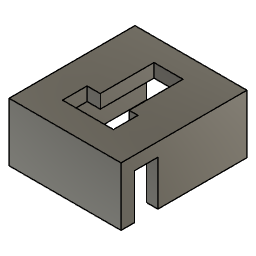
SNES - Back Cutting Tool v11 (Autodesk Fusion 360 design; units mm, degrees)
Autodesk Fusion 360 part; units mm, degrees
note: some values were not read from the file. Set by a fixed rule: which sketch regions a step uses.
sketch "Boceto1" plane through (0, 0, 0) normal (0, 0, 1) x (1, 0, 0)
  line L0 (4.725, 2.765) -> (4.725, -5.635)
  line L1 (4.725, -8.235) -> (-4.725, -8.235)
  line L2 (-4.725, -8.235) -> (-4.725, 2.765)
  line L3 (-6.225, 4.265) -> (6.225, 4.265)
  line L4 (6.225, 4.265) -> (6.225, -9.735)
  line L5 (6.225, -9.735) -> (-6.225, -9.735)
  line L6 (-6.225, -9.735) -> (-6.225, 4.265)
  line L7 (2.585, -4.215) -> (2.585, -6.945)
  line L8 (2.585, -6.945) -> (-3.075, -6.945)
  line L9 (-3.075, -6.945) -> (-3.075, -4.215)
  line L10 (-1.61, -4.215) -> (-1.61, 1.765)
  line L11 (1.61, 1.765) -> (1.61, -4.215)
  line L12 (-3.075, -4.215) -> (-1.61, -4.215)
  line L13 (1.61, -4.215) -> (2.585, -4.215)
  line L14 (-4.725, 2.765) -> (-4.725, 4.265)
  line L15 (4.725, 4.265) -> (4.725, 2.765)
  line L16 (4.725, -5.635) -> (6.225, -5.635)
  line L17 (4.725, -8.235) -> (6.225, -8.235)
  line L18 (-1.61, 1.765) -> (1.61, 1.765)
  dimension "d1" = 9.45
  dimension "d2" = 4.725
  dimension "d3" = 1.5
  dimension "d4" = 1.5
  dimension "d5" = 1.5
  dimension "d6" = 1.5
  dimension "d9" = 8.235
  dimension "d10" = 5.66
  dimension "d11" = 2.73
  dimension "d12" = 1.29
  dimension "d13" = 1.65
  dimension "d21" = 10
  dimension "d22" = 12.5
  dimension "d27" = 2.6
  dimension "d32" = 3.115
  dimension "d33" = 3.115
  constraint vertical L0
  constraint horizontal L1
  constraint vertical L2
  constraint horizontal L3
  constraint vertical L4
  constraint horizontal L5
  constraint vertical L6
  constraint horizontal L12
  constraint vertical L7
  constraint horizontal L8
  constraint vertical L9
  constraint perpendicular L10 L12
  constraint coincident L11.end L12
  constraint perpendicular L11 L12
  constraint collinear L12 L13
  constraint coincident L3 L14.end
  constraint perpendicular L3 L14
  constraint coincident L3 L15.start
  constraint coincident L4 L16.end
  constraint perpendicular L4 L16
  constraint coincident L4 L17.end
  constraint perpendicular L4 L17
  constraint perpendicular L11 L18
  measures "d1" distance of L2.end L0.start
  measures "d2" horizontal distance of origin L2.end
  measures "d3" horizontal distance of L2.end L3.start
  measures "d4" horizontal distance of L0.start L3.end
  measures "d5" vertical distance of L0.start L3.end
  measures "d6" vertical distance of L1.start L4.end
  measures "d9" vertical distance of origin L1.end
  measures "d10" distance of L9.end L7.start
  measures "d11" distance of L7.start L7.end
  measures "d12" vertical distance of L1.end L8.end
  measures "d13" horizontal distance of L1.end L8.end
  measures "d21" vertical distance of L1.end L10.end
  measures "d22" vertical distance of L1.end L3.start
  measures "d27" vertical distance of L1.start L16.end
  measures "d32" horizontal distance of L1.end L10.end
  measures "d33" horizontal distance of L11.start L15.start
extrude "Extruir5" add sketch "Boceto1" against normal blind 1.5 contours L0 L1 L2 L3 L4 L14 L15 L16 L17
extrude "Extruir6" add sketch "Boceto1" against normal blind 6.5 contours L0 L3 L4 L15 L16 | L1 L2 L3 L4 L5 L6 L14 L17
extrude "Extruir7" cut 1 faces at (-4.725, -4.0683, -3.1667) along direction (-1, 0, 0) blind 0.2
extrude "Extruir8" cut 1 faces at (4.725, 0.965, -3.1667) along direction (1, 0, 0) blind 0.2
equation "d2 = d1 / 2"
equation "d4 = d3"
equation "d5 = d3"
equation "d6 = d3"
equation "d7 = 16.47 mm"
equation "d9 = d7 / 2"
equation "d22 = d21 + d3 + 1 mm"
equation "d28 = -d3"
equation "d30 = -( d3 + 5 mm )"
equation "d32 = d1 / 2 - ( ( 3.22 / 2 ) * 1 mm )"
equation "d33 = d32"
